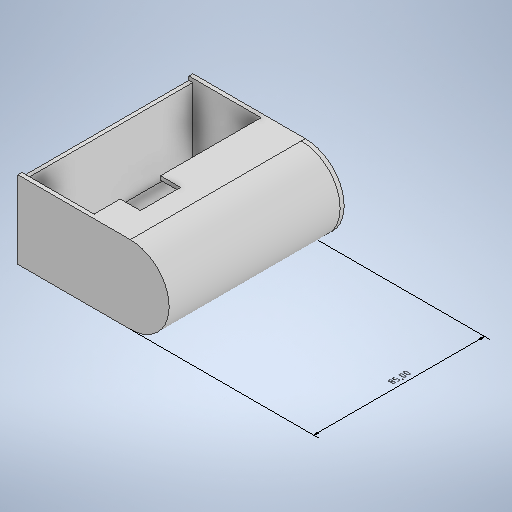
# Autodesk Inventor part: víko
Saved by Autodesk Inventor 2025.3 (Build 293356000, 356)
## iProperties
Created: 2025-06-12
Part Number: víko
Material: Generic
Document SubType Name: Modeling
Designer: Repete
Density: 1 g/cm^3
Appearance: Default
Author: Repete
Autodesk Inventor part; units mm, degrees
ref_plane "YZ Plane" through (0, 0, 0) normal (1, 0, 0) x (0, 1, 0)
ref_plane "XZ Plane" through (0, 0, 0) normal (0, 1, 0) x (-1, 0, 0)
ref_plane "XY Plane" through (0, 0, 0) normal (0, 0, 1) x (1, 0, 0)
sketch "Sketch1" plane through (0, 0, 0) normal (0, 1, 0) x (-1, 0, 0)
  line L0 (40.7987, 17.4) -> (40.7987, -17.4)
  line L1 (40.7987, -17.4) -> (-13.2013, -17.4)
  arc A0 (-13.2013, 17.4) -> (-13.2013, -17.4) centre (-13.2013, 0) ccw
  line L2 (-13.2013, 17.4) -> (40.7987, 17.4)
  line L3 (42.6987, -19.3) -> (42.6987, 19.3)
  line L4 (42.6987, 19.3) -> (-13.2013, 19.3)
  arc A1 (-13.2013, 19.3) -> (-13.2013, -19.3) centre (-13.2013, 0) ccw
  line L5 (-13.2013, -19.3) -> (42.6987, -19.3)
  point P0 (0, 0)
  point P1 (-13.2013, 0)
  point P2 (0, 0)
  point P3 (-12.8411, -36.7096)
  point P4 (-12.8411, -7.716)
  point P5 (-24.0253, -72.4098)
  dimension "d156" = 1.9
  dimension "d157" = 1.9
  dimension "d158" = 1.9
  dimension "d159" = 1.9
  dimension "d160" = 54
  constraints: 12 end point, 4 point on circle, 2 centre point, 2 parallel, 2 perpendicular
  measures "d156" distance between parallel lines of L3 L0
  measures "d157" distance between parallel lines of L2 L4
  measures "d158" distance between parallel lines of L5 L1
  measures "d159" radial gap between concentric circles of A1 A0
  measures "d160" distance from line of L0 A0.centre
extrude "Extrusion1" add sketch "Sketch1" along normal blind 83
ref_plane "Work Plane1" through (0, 85, 0) normal (0, 1, 0) x (1, 0, 0)
sketch "Sketch2" plane through (0, 85, 0) normal (0, 1, 0) x (1, 0, 0)
  line L0 (-42.6987, 19.3) -> (-42.6987, -19.3)
  line L1 (-42.6987, -19.3) -> (13.2164, -19.3)
  arc A0 (13.2164, -19.3) -> (13.2013, 19.3) centre (13.2013, 0) ccw
  line L2 (13.2013, 19.3) -> (-42.6987, 19.3)
  line L3 (-42.6987, 19.3) -> (-42.6987, -19.3) projected
  line L4 (-42.6987, -19.3) -> (13.2013, -19.3) projected
  arc A1 (13.2013, -19.3) -> (13.2013, 19.3) centre (13.2013, 0) ccw projected
  point P0 (0, 0)
  point P1 (14.0497, 95.3418)
  point P2 (14.0497, 124.3354)
  point P3 (2.8654, 59.6417)
  dimension "d163" = 38.6
  dimension "d165" = 19.3
  dimension "d166" = 0
  dimension "d167" = 0
  dimension "d168" = 0
  constraints: 6 end point, 2 point on circle, 1 centre point, 1 parallel, 1 perpendicular
  measures "d163" distance between parallel lines of L2 L1
  measures "d165" radius of A0
  measures "d166" distance between parallel lines of L4 L1
  measures "d167" distance between parallel lines of L3 L0
  measures "d168" distance of A1.centre A0.centre
extrude "Extrusion2" add sketch "Sketch2" against normal up to surface (2 mm away)
ref_plane "Work Plane2" through (-42.6987, 0, 19.3) normal (0, -1, 0) x (1, 0, 0)
sketch "Sketch35" plane through (-42.6987, 0, 19.3) normal (0, -1, 0) x (1, 0, 0)
  line L0 (0, 0) -> (0, -38.6)
  line L1 (0, -38.6) -> (55.9, -38.6)
  arc A0 (55.9, -38.6) -> (55.9, 0) centre (55.9, -19.3) ccw
  line L2 (55.9, 0) -> (0, 0)
  line L3 (0, 0) -> (55.9, 0) projected
  arc A1 (55.9, -38.6) -> (55.9, 0) centre (55.9, -19.3) ccw projected
  line L4 (0, -38.6) -> (0, 0) projected
  point P0 (17.1629, -27.1873)
  point P1 (30.3642, -27.1873)
  point P2 (17.1629, -27.1873)
  point P3 (14.0497, 95.3418)
  point P4 (14.0497, 124.3354)
  point P5 (2.8654, 59.6417)
  dimension "d132" = 19.3
  dimension "d133" = 0
  dimension "d162" = 0
  constraints: 6 end point, 2 point on circle, 1 centre point, 1 parallel, 1 perpendicular
  measures "d132" radius of A0
  measures "d133" radial gap between concentric circles of A1 A0
  measures "d162" distance between parallel lines of L4 L0
extrude "Extrusion24" add sketch "Sketch35" along normal blind 2
sketch "Sketch37" plane through (-42.6987, 85, 19.3) normal (0, 0, 1) x (1, 0, 0)
  line L0 (35.9, -85) -> (0, -85)
  line L1 (0, -85) -> (0, -2)
  line L2 (0, -2) -> (35.9, -2)
  line L3 (35.9, -2) -> (35.9, -85)
  line L4 (55.9, -85) -> (1.9, -85) projected
  line L5 (55.9, -2) -> (1.9, -2) projected
  line L6 (0, 0) -> (0, -87) projected
  line L7 (55.9, -87) -> (55.9, 0) projected
  point P0 (42.6987, -85)
  point P1 (55.9151, 0)
  dimension "d143" = 0
  dimension "d144" = 0
  dimension "d145" = 0
  dimension "d146" = 20
  constraints: 8 end point, 2 parallel, 1 horizontal, 1 perpendicular, 1 other
  measures "d143" distance between parallel lines of L4 L0
  measures "d144" distance between parallel lines of L5 L2
  measures "d145" distance between parallel lines of L6 L1
extrude "Extrusion26" cut sketch "Sketch37" against normal up to surface (1.9 mm away) contours L0 L1 L2 L3
sketch "Sketch38" plane through (-42.6987, 85, 19.3) normal (0, 0, 1) x (1, 0, 0)
  line L0 (35.9, -85) -> (35.9, -2) projected
  line L1 (45.9, -72) -> (35.9, -72)
  line L2 (35.9, -72) -> (35.9, -52)
  line L3 (35.9, -52) -> (45.9, -52)
  line L4 (45.9, -52) -> (45.9, -72)
  line L5 (55.9, -87) -> (0, -87) projected
  point P0 (42.6987, -85)
  point P1 (35.9, -72)
  dimension "d149" = 20
  dimension "d150" = 10
  dimension "d151" = 15
  constraints: 8 end point, 2 parallel, 1 horizontal, 1 perpendicular, 1 point on line
  measures "d149" distance between parallel lines of L3 L1
  measures "d150" distance between parallel lines of L0 L4
  measures "d151" distance between parallel lines of L1 L5
extrude "Extrusion27" cut sketch "Sketch38" against normal up to surface (1.9 mm away)
body "Solid1"
